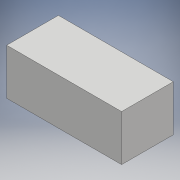
# Autodesk Inventor part: Side pontoon2
Saved by Autodesk Inventor 2018 (Build 220112000, 112)
## iProperties
Created: 2018-02-19
Part Number: Side pontoon2
Material: 一般
Document SubType Name: Modeling
Designer: kit
Density: 1 g/cm^3
Appearance: 既定
Author: kit
Autodesk Inventor part; units mm, degrees
ref_plane "YZ Plane" through (0, 0, 0) normal (1, 0, 0) x (0, 1, 0)
ref_plane "XZ Plane" through (0, 0, 0) normal (0, 1, 0) x (-1, 0, 0)
ref_plane "XY Plane" through (0, 0, 0) normal (0, 0, 1) x (1, 0, 0)
sketch "スケッチ1" plane through (0, 0, 0) normal (1, 0, 0) x (0, 1, 0)
  line L0 (-371.0199, 146.2166) -> (-821.0199, 146.2166)
  line L1 (-821.0199, 146.2166) -> (-821.0199, -253.7834)
  line L2 (-821.0199, -253.7834) -> (-371.0199, -253.7834)
  line L3 (-371.0199, -253.7834) -> (-371.0199, 146.2166)
  point P0 (0, 0)
  dimension "d2" = 400
  dimension "d3" = 450
  constraints: 8 end point, 2 parallel, 1 horizontal, 1 perpendicular
  measures "d2" distance of L2.end L0.start
  measures "d3" distance of L0.start L0.end
extrude "押し出し1" add sketch "スケッチ1" along normal blind 1000
